Autodesk Fusion 360 part; units mm, degrees
note: some values were not read from the file. Chosen so that the rebuilt part matches the saved one: that a step has no effect.
(part 5 of 7)
  spline S1394 degree 3 poles (-52.4461, -9.6584) (-55.3128, -12.1512) (-55.3128, -12.1512) (-56.4346, -12.1512) knots 0 0 0 0 1 1 1 1
  spline S1395 degree 3 poles (-56.4346, -12.1512) (-56.0918, -10.9671) (-56.0918, -10.9671) (-55.4375, -9.6584) knots 0 0 0 0 1 1 1 1
  spline S1396 degree 3 poles (-55.4375, -9.6584) (-54.1287, -9.0041) (-54.1287, -9.0041) (-52.9447, -8.6613) knots 0 0 0 0 1 1 1 1
  spline S1397 degree 3 poles (11.369, -4.6729) (11.6981, -4.6729) (12.0271, -4.6729) (12.3662, -4.6729) knots 0 0 0 0 1 1 1 1
  spline S1398 degree 3 poles (12.3662, -4.6729) (12.2259, -5.4113) (12.0793, -6.1486) (11.9299, -6.8852) knots 0 0 0 0 1 1 1 1
  spline S1399 degree 3 poles (11.9299, -6.8852) (11.8489, -7.2959) (11.768, -7.7065) (11.6845, -8.1297) knots 0 0 0 0 1 1 1 1
  spline S1400 degree 3 poles (11.6845, -8.1297) (11.5284, -8.6396) (11.5284, -8.6396) (11.369, -9.1599) knots 0 0 0 0 1 1 1 1
  spline S1401 degree 3 poles (11.369, -9.1599) (10.8755, -9.4067) (10.8755, -9.4067) (10.3719, -9.6584) knots 0 0 0 0 1 1 1 1
  spline S1402 degree 3 poles (10.3719, -9.6584) (10.2825, -7.6905) (10.3253, -6.3689) (11.369, -4.6729) knots 0 0 0 0 1 1 1 1
  spline S1403 degree 3 poles (-34.4981, 8.2896) (-34.0045, 8.2896) (-33.511, 8.2896) (-33.0024, 8.2896) knots 0 0 0 0 1 1 1 1
  spline S1404 degree 3 poles (-33.0024, 8.2896) (-32.5039, 6.7939) (-32.5039, 6.7939) (-33.2206, 5.2048) knots 0 0 0 0 1 1 1 1
  spline S1405 degree 3 poles (-33.2206, 5.2048) (-33.6062, 4.5107) (-33.6062, 4.5107) (-33.9995, 3.8026) knots 0 0 0 0 1 1 1 1
  spline S1406 degree 3 poles (-33.9995, 3.8026) (-34.1641, 3.8026) (-34.3286, 3.8026) (-34.4981, 3.8026) knots 0 0 0 0 1 1 1 1
  spline S1407 degree 3 poles (-34.4981, 3.8026) (-34.9363, 6.8699) (-34.9363, 6.8699) (-34.9967, 7.791) knots 0 0 0 0 1 1 1 1
  spline S1408 degree 3 poles (-34.9967, 7.791) (-34.8321, 7.9556) (-34.6676, 8.1201) (-34.4981, 8.2896) knots 0 0 0 0 1 1 1 1
  spline S1409 degree 3 poles (-20.5385, 11.2809) (-20.374, 11.2809) (-20.2095, 11.2809) (-20.04, 11.2809) knots 0 0 0 0 1 1 1 1
  spline S1410 degree 3 poles (-20.04, 11.2809) (-20.04, 9.9647) (-20.04, 8.6485) (-20.04, 7.2925) knots 0 0 0 0 1 1 1 1
  spline S1411 degree 3 poles (-20.04, 7.2925) (-20.369, 7.2925) (-20.6981, 7.2925) (-21.0371, 7.2925) knots 0 0 0 0 1 1 1 1
  spline S1412 degree 3 poles (-21.0371, 7.2925) (-21.2016, 6.9634) (-21.3661, 6.6344) (-21.5356, 6.2954) knots 0 0 0 0 1 1 1 1
  spline S1413 degree 3 poles (-21.5356, 6.2954) (-21.7002, 6.9535) (-21.8647, 7.6116) (-22.0342, 8.2896) knots 0 0 0 0 1 1 1 1
  spline S1414 degree 3 poles (-22.0342, 8.2896) (-21.7052, 8.2896) (-21.3761, 8.2896) (-21.0371, 8.2896) knots 0 0 0 0 1 1 1 1
  spline S1415 degree 3 poles (-21.0371, 8.2896) (-21.0525, 8.8911) (-21.0525, 8.8911) (-21.0683, 9.5048) knots 0 0 0 0 1 1 1 1
  spline S1416 degree 3 poles (-21.0683, 9.5048) (-21.0371, 10.7824) (-21.0371, 10.7824) (-20.5385, 11.2809) knots 0 0 0 0 1 1 1 1
  spline S1417 degree 3 poles (0.8994, 35.2116) (1.0639, 35.2116) (1.2284, 35.2116) (1.3979, 35.2116) knots 0 0 0 0 1 1 1 1
  spline S1418 degree 3 poles (1.3979, 35.2116) (1.5624, 33.8954) (1.727, 32.5792) (1.8965, 31.2232) knots 0 0 0 0 1 1 1 1
  spline S1419 degree 3 poles (1.8965, 31.2232) (1.2384, 31.0586) (0.5803, 30.8941) (-0.0977, 30.7246) knots 0 0 0 0 1 1 1 1
  spline S1420 degree 3 poles (-0.0977, 30.7246) (0.2313, 32.2053) (0.5604, 33.686) (0.8994, 35.2116) knots 0 0 0 0 1 1 1 1
  spline S1421 degree 3 poles (31.3113, 37.2058) (31.4758, 36.7123) (31.6403, 36.2187) (31.8098, 35.7102) knots 0 0 0 0 1 1 1 1
  spline S1422 degree 3 poles (31.8098, 35.7102) (30.1808, 32.9014) (30.1808, 32.9014) (28.8185, 32.2203) knots 0 0 0 0 1 1 1 1
  spline S1423 degree 3 poles (28.8185, 32.2203) (29.0709, 34.0878) (29.3957, 34.9688) (30.8127, 36.2087) knots 0 0 0 0 1 1 1 1
  spline S1424 degree 3 poles (30.8127, 36.2087) (30.9773, 36.5378) (31.1418, 36.8668) (31.3113, 37.2058) knots 0 0 0 0 1 1 1 1
  spline S1425 degree 3 poles (-1.5934, 42.69) (-1.5934, 42.0319) (-1.5934, 41.3738) (-1.5934, 40.6957) knots 0 0 0 0 1 1 1 1
  spline S1426 degree 3 poles (-1.5934, 40.6957) (-1.9225, 40.6957) (-2.2515, 40.6957) (-2.5905, 40.6957) knots 0 0 0 0 1 1 1 1
  spline S1427 degree 3 poles (-2.5905, 40.6957) (-2.755, 40.2022) (-2.9196, 39.7086) (-3.0891, 39.2001) knots 0 0 0 0 1 1 1 1
  spline S1428 degree 3 poles (-3.0891, 39.2001) (-3.5876, 39.6986) (-3.5876, 39.6986) (-3.6188, 40.9762) knots 0 0 0 0 1 1 1 1
  spline S1429 degree 3 poles (-3.6188, 40.9762) (-3.6085, 41.3772) (-3.5982, 41.7782) (-3.5876, 42.1914) knots 0 0 0 0 1 1 1 1
  spline S1430 degree 3 poles (-3.5876, 42.1914) (-2.5905, 42.69) (-2.5905, 42.69) (-1.5934, 42.69) knots 0 0 0 0 1 1 1 1
  spline S1431 degree 3 poles (-77.3739, 6.2954) (-77.2094, 6.2954) (-77.0449, 6.2954) (-76.8754, 6.2954) knots 0 0 0 0 1 1 1 1
  spline S1432 degree 3 poles (-76.8754, 6.2954) (-77.0399, 4.4856) (-77.2044, 2.6758) (-77.3739, 0.8112) knots 0 0 0 0 1 1 1 1
  spline S1433 degree 3 poles (-77.3739, 0.8112) (-77.5384, 0.8112) (-77.703, 0.8112) (-77.8725, 0.8112) knots 0 0 0 0 1 1 1 1
  spline S1434 degree 3 poles (-77.8725, 0.8112) (-78.4861, 4.002) (-78.4861, 4.002) (-77.9036, 5.5164) knots 0 0 0 0 1 1 1 1
  spline S1435 degree 3 poles (-77.9036, 5.5164) (-77.7288, 5.7734) (-77.554, 6.0305) (-77.3739, 6.2954) knots 0 0 0 0 1 1 1 1
  spline S1436 degree 3 poles (-4.0862, 5.2983) (-3.5926, 5.2983) (-3.099, 5.2983) (-2.5905, 5.2983) knots 0 0 0 0 1 1 1 1
  spline S1437 degree 3 poles (-2.5905, 5.2983) (-2.7152, 4.1142) (-2.7152, 4.1142) (-3.0891, 2.8055) knots 0 0 0 0 1 1 1 1
  spline S1438 degree 3 poles (-3.0891, 2.8055) (-4.1173, 2.1511) (-4.1173, 2.1511) (-5.0833, 1.8084) knots 0 0 0 0 1 1 1 1
  spline S1439 degree 3 poles (-5.0833, 1.8084) (-4.7543, 2.96) (-4.4252, 4.1117) (-4.0862, 5.2983) knots 0 0 0 0 1 1 1 1
  spline S1440 degree 3 poles (18.3488, 14.7708) (18.1843, 13.9482) (18.0198, 13.1256) (17.8503, 12.278) knots 0 0 0 0 1 1 1 1
  spline S1441 degree 3 poles (17.8503, 12.278) (17.3567, 12.4426) (16.8631, 12.6071) (16.3546, 12.7766) knots 0 0 0 0 1 1 1 1
  spline S1442 degree 3 poles (16.3546, 12.7766) (16.1901, 13.2702) (16.0256, 13.7637) (15.8561, 14.2723) knots 0 0 0 0 1 1 1 1
  spline S1443 degree 3 poles (15.8561, 14.2723) (16.8532, 14.7708) (16.8532, 14.7708) (18.3488, 14.7708) knots 0 0 0 0 1 1 1 1
  spline S1444 degree 3 poles (-68.8985, 21.7506) (-68.5694, 21.7506) (-68.2404, 21.7506) (-67.9014, 21.7506) knots 0 0 0 0 1 1 1 1
  spline S1445 degree 3 poles (-67.9014, 21.7506) (-68.546, 20.3126) (-69.2272, 19.3215) (-70.3941, 18.2607) knots 0 0 0 0 1 1 1 1
  spline S1446 degree 3 poles (-70.3941, 18.2607) (-70.7232, 18.4252) (-71.0522, 18.5898) (-71.3913, 18.7593) knots 0 0 0 0 1 1 1 1
  spline S1447 degree 3 poles (-71.3913, 18.7593) (-70.5856, 19.7769) (-69.7532, 20.7738) (-68.8985, 21.7506) knots 0 0 0 0 1 1 1 1
  spline S1448 degree 3 poles (-7.5761, 35.2116) (-6.918, 35.0471) (-6.2599, 34.8826) (-5.5819, 34.7131) knots 0 0 0 0 1 1 1 1
  spline S1449 degree 3 poles (-5.5819, 34.7131) (-5.5819, 34.055) (-5.5819, 33.3969) (-5.5819, 32.7188) knots 0 0 0 0 1 1 1 1
  spline S1450 degree 3 poles (-5.5819, 32.7188) (-6.24, 32.7188) (-6.898, 32.7188) (-7.5761, 32.7188) knots 0 0 0 0 1 1 1 1
  spline S1451 degree 3 poles (-7.5761, 32.7188) (-7.5761, 33.5414) (-7.5761, 34.3641) (-7.5761, 35.2116) knots 0 0 0 0 1 1 1 1
  spline S1452 degree 3 poles (-45.9649, -7.6642) (-45.6358, -8.1578) (-45.3068, -8.6513) (-44.9678, -9.1599) knots 0 0 0 0 1 1 1 1
  spline S1453 degree 3 poles (-44.9678, -9.1599) (-45.4614, -9.4067) (-45.4614, -9.4067) (-45.9649, -9.6584) knots 0 0 0 0 1 1 1 1
  spline S1454 degree 3 poles (-45.9649, -9.6584) (-46.29, -10.6678) (-46.29, -10.6678) (-46.4635, -11.6527) knots 0 0 0 0 1 1 1 1
  spline S1455 degree 3 poles (-46.4635, -11.6527) (-46.957, -11.6527) (-47.4506, -11.6527) (-47.9591, -11.6527) knots 0 0 0 0 1 1 1 1
  spline S1456 degree 3 poles (-47.9591, -11.6527) (-47.3985, -10.171) (-46.8509, -8.9932) (-45.9649, -7.6642) knots 0 0 0 0 1 1 1 1
  spline S1457 degree 3 poles (-27.0198, -8.6613) (-26.5262, -8.6613) (-26.0326, -8.6613) (-25.5241, -8.6613) knots 0 0 0 0 1 1 1 1
  spline S1458 degree 3 poles (-25.5241, -8.6613) (-25.5241, -9.6485) (-25.5241, -10.6356) (-25.5241, -11.6527) knots 0 0 0 0 1 1 1 1
  spline S1459 degree 3 poles (-25.5241, -11.6527) (-26.0177, -11.6527) (-26.5112, -11.6527) (-27.0198, -11.6527) knots 0 0 0 0 1 1 1 1
  spline S1460 degree 3 poles (-27.0198, -11.6527) (-27.0198, -10.6655) (-27.0198, -9.6784) (-27.0198, -8.6613) knots 0 0 0 0 1 1 1 1
  spline S1461 degree 3 poles (32.3084, 31.7217) (33.2955, 31.4749) (33.2955, 31.4749) (34.3026, 31.2232) knots 0 0 0 0 1 1 1 1
  spline S1462 degree 3 poles (34.3026, 31.2232) (34.3026, 30.5651) (34.3026, 29.907) (34.3026, 29.2289) knots 0 0 0 0 1 1 1 1
  spline S1463 degree 3 poles (34.3026, 29.2289) (33.48, 29.3935) (32.6574, 29.558) (31.8098, 29.7275) knots 0 0 0 0 1 1 1 1
  spline S1464 degree 3 poles (31.8098, 29.7275) (32.3034, 30.2211) (32.797, 30.7146) (33.3055, 31.2232) knots 0 0 0 0 1 1 1 1
  spline S1465 degree 3 poles (33.3055, 31.2232) (32.9765, 31.3877) (32.6474, 31.5522) (32.3084, 31.7217) knots 0 0 0 0 1 1 1 1
sketch "Sketch84" plane through (76.6406, 0, 0) normal (1, 0, 0) x (0, 1, 0)
  line L0 (66.6352, 16.8343) -> (66.6352, 146.8343)
  line L1 (66.6352, 146.8343) -> (-58.3648, 111.8343)
  line L2 (-58.3648, 16.8343) -> (66.6352, 16.8343)
sketch "Sketch85" plane through (0, 0, 0) normal (1, 0, 0) x (0, 1, 0)
sketch "Sketch86" plane through (76.6406, 0, 0) normal (1, 0, 0) x (0, 1, 0)
sketch "Sketch87" plane through (76.6406, 0, 0) normal (1, 0, 0) x (0, 1, 0)
sketch "Sketch88" plane through (0, 0, 0) normal (0, 1, 0) x (1, 0, 0)
  line L0 (76.6406, -111.8343) -> (-103.3594, -111.8343)
  line L1 (-103.3594, -111.8343) -> (-103.3594, -16.8343)
  line L2 (-103.3594, -16.8343) -> (76.6406, -16.8343)
  line L3 (76.6406, -111.8343) -> (76.6406, -16.8343)
  line L4 (-103.3594, -111.8343) -> (76.6406, -111.8343)
  line L5 (76.6406, -111.8343) -> (76.6406, -16.8343)
  line L6 (76.6406, -16.8343) -> (-103.3594, -16.8343)
  line L7 (-103.3594, -16.8343) -> (-103.3594, -111.8343)
  constraint horizontal L4
  constraint vertical L5
  constraint horizontal L6
  constraint vertical L7
  constraint coincident L2.end L3.end
  constraint coincident L0.end L1.start
copy_body "Body->Comp1" bodies 1 removing the originals makes body 2 in component "Component"
sketch "Sketch89" plane through (-3.3594, 0, 0) normal (-1, 0, 0) x (0, -1, 0)
  line L0 (58.3648, 39.3343) -> (58.3648, 86.8343)
  line L1 (58.3648, 86.8343) -> (53.3648, 86.8343)
  line L2 (53.3648, 86.8343) -> (53.3648, 39.3343)
  line L3 (53.3648, 39.3343) -> (58.3648, 39.3343)
  line L4 (53.3648, 39.3343) -> (53.3648, 108.042)
  line L5 (58.3648, 111.8343) -> (58.3648, 16.8343)
  line L6 (58.3648, 39.3343) -> (53.3648, 39.3343)
  line L7 (57.3648, 39.3343) -> (54.3648, 39.3343)
  line L8 (54.3648, 39.3343) -> (54.3648, 64.7338)
  line L9 (54.3648, 64.7338) -> (57.3648, 64.7338)
  line L10 (57.3648, 64.7338) -> (57.3648, 39.3343)
  dimension "d135" = 3
  dimension "d136" = 1
  constraint horizontal L7
  constraint vertical L8
  constraint horizontal L9
  constraint vertical L10
  constraint coincident L3 L7.start
  measures "d135" distance of L7.start L7.end
  measures "d136" distance of L4 L8
extrude "Extrude1" cut sketch "Sketch89" along normal blind 95 and the other way blind 75 contours L3 L6 L7 L8 L9 L10 bodies 2 in component "Component"
sketch "Sketch90" plane through (-3.3594, 0, 0) normal (-1, 0, 0) x (0, -1, 0)
  line L0 (54.3648, 39.3343) -> (54.3648, 64.7338)
  line L1 (54.3648, 64.7338) -> (57.3648, 64.7338)
  line L2 (57.3648, 64.7338) -> (57.3648, 39.3343)
  line L3 (57.3648, 39.3343) -> (58.3648, 39.3343)
  line L4 (58.3648, 39.3343) -> (58.3648, 86.8343)
  line L5 (58.3648, 86.8343) -> (53.3648, 86.8343)
  line L6 (53.3648, 86.8343) -> (53.3648, 39.3343)
  line L7 (53.3648, 39.3343) -> (54.3648, 39.3343)
sketch "Sketch91" plane through (0, -58.3648, 0) normal (0, -1, 0) x (1, 0, 0)
  line L0 (-23.3594, 39.3343) -> (-23.3594, 86.8343)
  arc A0 (-3.3594, 86.8343) -> (-23.3594, 86.8343) centre (-13.3594, 86.8343) ccw
  line L1 (-3.3594, 86.8343) -> (-3.3594, 39.3343)
  line L2 (-3.3594, 39.3343) -> (71.6406, 39.3343)
  line L3 (71.6406, 39.3343) -> (71.6406, 16.8343)
  line L4 (71.6406, 16.8343) -> (76.6406, 16.8343)
  line L5 (76.6406, 16.8343) -> (76.6406, 111.8343)
  line L6 (76.6406, 111.8343) -> (-103.3594, 111.8343)
  line L7 (-103.3594, 111.8343) -> (-103.3594, 16.8343)
  line L8 (-103.3594, 16.8343) -> (-98.3594, 16.8343)
  line L9 (-98.3594, 16.8343) -> (-98.3594, 39.3343)
  line L10 (-98.3594, 39.3343) -> (-23.3594, 39.3343)
  line L11 (7, 75) -> (-31, 75)
  line L12 (-31, 75) -> (-31, 101)
  line L13 (-31, 101) -> (7, 101)
  line L14 (7, 101) -> (7, 75)
  constraint horizontal L11
  constraint vertical L12
  constraint horizontal L13
  constraint vertical L14
extrude "Extrude2" add sketch "Sketch91" against normal blind 5 contours L0 A0 L1 L11 bodies 2 in component "Component"
sketch "Sketch92" plane through (-3.3594, 0, 0) normal (-1, 0, 0) x (0, -1, 0)
  line L0 (53.3648, 86.8343) -> (53.3648, 39.3343)
  line L1 (58.3648, 111.8343) -> (58.3648, 16.8343)
  line L2 (57.3648, 64.3343) -> (54.3648, 64.3343)
  line L3 (54.3648, 64.3343) -> (54.3648, 91)
  line L4 (54.3648, 91) -> (57.3648, 91)
  line L5 (57.3648, 91) -> (57.3648, 64.3343)
  dimension "d143" = 3
  dimension "d144" = 1
  constraint horizontal L2
  constraint vertical L3
  constraint horizontal L4
  constraint vertical L5
  measures "d143" distance of L2.start L2.end
  measures "d144" distance of L0 L3
extrude "Extrude3" cut sketch "Sketch92" along normal blind 95 and the other way blind 75 bodies 2 in component "Component"
sketch "Sketch93" plane through (0, -58.3648, 0) normal (0, -1, 0) x (1, 0, 0)
  line L0 (-23.3594, 39.3343) -> (-23.3594, 75)
  line L1 (-23.3594, 75) -> (-3.3594, 75)
  line L2 (-3.3594, 75) -> (-3.3594, 39.3343)
  line L3 (-3.3594, 39.3343) -> (71.6406, 39.3343)
  line L4 (71.6406, 39.3343) -> (71.6406, 16.8343)
  line L5 (71.6406, 16.8343) -> (76.6406, 16.8343)
  line L6 (76.6406, 16.8343) -> (76.6406, 111.8343)
  line L7 (76.6406, 111.8343) -> (-103.3594, 111.8343)
  line L8 (-103.3594, 111.8343) -> (-103.3594, 16.8343)
  line L9 (-103.3594, 16.8343) -> (-98.3594, 16.8343)
  line L10 (-98.3594, 16.8343) -> (-98.3594, 39.3343)
  line L11 (-98.3594, 39.3343) -> (-23.3594, 39.3343)
  line L12 (-3.3594, 39.3343) -> (-3.3594, 86.8343)
  line L13 (-3.3594, 75) -> (-23.3594, 75)
  line L14 (-23.3594, 39.3343) -> (-23.3594, 75)
  line L15 (-98.3594, 39.3343) -> (-23.3594, 39.3343)
  line L16 (-3.3594, 39.3343) -> (71.6406, 39.3343)
  line L17 (-98.3594, 16.8343) -> (-98.3594, 39.3343)
  line L18 (71.6406, 21.8343) -> (-98.3594, 21.8343)
  line L19 (71.6406, 16.8343) -> (71.6406, 39.3343)
  line L20 (-23.3594, 75) -> (-3.3594, 75)
  line L21 (-3.3594, 75) -> (-3.3594, 39.3343)
  line L22 (-3.3594, 39.3343) -> (-23.3594, 39.3343)
  line L23 (-23.3594, 39.3343) -> (-23.3594, 75)
  line L24 (-98.3594, 39.3343) -> (71.6406, 39.3343)
  line L25 (71.6406, 39.3343) -> (71.6406, 18.7368)
  line L26 (71.6406, 18.7368) -> (-98.3594, 18.7368)
  line L27 (-98.3594, 18.7368) -> (-98.3594, 39.3343)
  constraint horizontal L20
  constraint vertical L21
  constraint horizontal L22
  constraint vertical L23
  constraint coincident L2.end L3.start
  constraint coincident L0.end L1.start
  constraint horizontal L24
  constraint vertical L25
  constraint horizontal L26
  constraint vertical L27
  constraint coincident L19 L25.end
  constraint coincident L10.end L11.start
sketch "Sketch94" plane through (0, -61.3648, 0) normal (0, -1, 0) x (1, 0, 0)
sketch "Sketch95" plane through (0, -61.3648, 0) normal (0, -1, 0) x (1, 0, 0)
  line L0 (-23.3594, 75) -> (-23.3594, 39.3343)
  line L1 (-3.3594, 39.3343) -> (-3.3594, 75)
  line L2 (-3.3594, 71.6642) -> (-23.3594, 71.6642)
  line L3 (-23.3594, 71.6642) -> (-23.3594, 81.6642)
  line L4 (-23.3594, 81.6642) -> (-3.3594, 81.6642)
  line L5 (-3.3594, 81.6642) -> (-3.3594, 71.6642)
  dimension "d151" = 20
  dimension "d152" = 10
  constraint horizontal L2
  constraint vertical L3
  constraint horizontal L4
  constraint vertical L5
  constraint coincident L1 L2.start
  measures "d151" distance of L2.start L2.end
  measures "d152" distance of L2.start L4.end
sketch "Sketch96" plane through (0, 0, 0) normal (1, 0, 0) x (0, 1, 0)
fillet "Fillet1" radius 5 1 edges at (-13.3594, 66.6352, 146.8343) on bodies 2 in component "Component"
fillet "Fillet2'" radius 7.5 1 edges at (-13.3594, -58.3648, 111.8343) on bodies 2 in component "Component"
sketch "Sketch97" plane through (0, -58.3648, 0) normal (0, -1, 0) x (1, 0, 0)
  line L0 (76.6406, 106.1458) -> (-103.3594, 106.1458)
  line L1 (-103.3594, 106.1458) -> (-103.3594, 16.8343)
  line L2 (-103.3594, 16.8343) -> (-98.3594, 16.8343)
  line L3 (-98.3594, 16.8343) -> (-98.3594, 39.3343)
  line L4 (-98.3594, 39.3343) -> (-23.3594, 39.3343)
  line L5 (-23.3594, 39.3343) -> (-23.3594, 75)
  line L6 (-23.3594, 75) -> (-3.3594, 75)
  line L7 (-3.3594, 39.3343) -> (71.6406, 39.3343)
  line L8 (71.6406, 16.8343) -> (76.6406, 16.8343)
  line L9 (76.6406, 16.8343) -> (76.6406, 106.1458)
sketch "Sketch98" plane through (71.6406, 0, 0) normal (-1, 0, 0) x (0, -1, 0)
  arc A0 (-60.2871, 145.0568) -> (-61.6142, 145.2419) centre (-61.6352, 140.242) ccw
  arc A1 (-61.6142, 145.2419) -> (10.7755, 21.8343) centre (112.3399, 164.3463) ccw
  line L0 (10.7755, 21.8343) -> (46.1173, 21.8343)
  arc A2 (58.3648, 16.8343) -> (46.1173, 21.8343) centre (46.1173, 4.3343) ccw
  line L1 (58.3648, 16.8343) -> (58.3648, 39.3343)
  line L2 (58.3648, 39.3343) -> (57.3648, 39.3343)
  line L3 (57.3648, 39.3343) -> (57.3648, 91)
  line L4 (57.3648, 91) -> (54.3648, 91)
  line L5 (54.3648, 91) -> (54.3648, 39.3343)
  line L6 (54.3648, 39.3343) -> (53.3648, 39.3343)
  line L7 (53.3648, 39.3343) -> (53.3648, 108.042)
  line L8 (53.3648, 108.042) -> (-27.8352, 130.778)
  line L9 (-27.8352, 130.778) -> (-26.4871, 135.5928)
  line L10 (-26.4871, 135.5928) -> (-60.2871, 145.0568)
sketch "Sketch99" plane through (71.6406, 0, 0) normal (-1, 0, 0) x (0, -1, 0)
sketch "Sketch100" plane through (-103.3594, 0, 0) normal (-1, 0, 0) x (0, -1, 0)
  arc A0 (58.3648, 106.1458) -> (52.887, 113.3681) centre (50.8648, 106.1458) ccw
  line L0 (52.887, 113.3681) -> (-60.2871, 145.0568)
  arc A1 (-60.2871, 145.0568) -> (-66.6352, 140.242) centre (-61.6352, 140.242) ccw
  line L1 (-66.6352, 140.242) -> (-66.6352, 16.8343)
  line L2 (-66.6352, 16.8343) -> (58.3648, 16.8343)
  line L3 (58.3648, 16.8343) -> (58.3648, 106.1458)
  spline S0 degree 3 poles (2.2852, 67.0349) (2.2852, 66.9197) (2.2852, 66.8045) (2.2852, 66.6858) knots 0 0 0 0 1 1 1 1
  spline S1 degree 3 poles (2.2852, 66.6858) (2.3869, 66.6426) (2.4886, 66.5994) (2.5934, 66.5549) knots 0 0 0 0 1 1 1 1
  spline S2 degree 3 poles (2.5934, 66.5549) (3.0411, 66.3044) (3.304, 66.0266) (3.6379, 65.6385) knots 0 0 0 0 1 1 1 1
  spline S3 degree 3 poles (3.6379, 65.6385) (3.7985, 65.4549) (3.7985, 65.4549) (3.9624, 65.2676) knots 0 0 0 0 1 1 1 1
  spline S4 degree 3 poles (3.9624, 65.2676) (4.2052, 64.9404) (4.2052, 64.9404) (4.2052, 64.5913) knots 0 0 0 0 1 1 1 1
  spline S5 degree 3 poles (4.2052, 64.5913) (4.3204, 64.5913) (4.4356, 64.5913) (4.5543, 64.5913) knots 0 0 0 0 1 1 1 1
  spline S6 degree 3 poles (4.5543, 64.5913) (4.8188, 64.3165) (4.8188, 64.3165) (5.1215, 63.9476) knots 0 0 0 0 1 1 1 1
  spline S7 degree 3 poles (5.1215, 63.9476) (5.5144, 63.4823) (5.8983, 63.071) (6.3761, 62.6931) knots 0 0 0 0 1 1 1 1
  spline S8 degree 3 poles (6.3761, 62.6931) (6.5237, 62.5707) (6.6713, 62.4483) (6.8233, 62.3222) knots 0 0 0 0 1 1 1 1
  spline S9 degree 3 poles (6.8233, 62.3222) (6.8233, 62.207) (6.8233, 62.0918) (6.8233, 61.9731) knots 0 0 0 0 1 1 1 1
  spline S10 degree 3 poles (6.8233, 61.9731) (6.9385, 61.9731) (7.0537, 61.9731) (7.1724, 61.9731) knots 0 0 0 0 1 1 1 1
  spline S11 degree 3 poles (7.1724, 61.9731) (7.1724, 61.8579) (7.1724, 61.7427) (7.1724, 61.624) knots 0 0 0 0 1 1 1 1
  spline S12 degree 3 poles (7.1724, 61.624) (7.2876, 61.624) (7.4028, 61.624) (7.5215, 61.624) knots 0 0 0 0 1 1 1 1
  spline S13 degree 3 poles (7.5215, 61.624) (7.5215, 61.5088) (7.5215, 61.3936) (7.5215, 61.2749) knots 0 0 0 0 1 1 1 1
  spline S14 degree 3 poles (7.5215, 61.2749) (7.6196, 61.2299) (7.7177, 61.1849) (7.8188, 61.1385) knots 0 0 0 0 1 1 1 1
  spline S15 degree 3 poles (7.8188, 61.1385) (8.2663, 60.9011) (8.6477, 60.6242) (9.0488, 60.3149) knots 0 0 0 0 1 1 1 1
  spline S16 degree 3 poles (9.0488, 60.3149) (9.258, 60.1556) (9.258, 60.1556) (9.4715, 59.9931) knots 0 0 0 0 1 1 1 1
  spline S17 degree 3 poles (9.4715, 59.9931) (9.5768, 59.8977) (9.6821, 59.8023) (9.7906, 59.704) knots 0 0 0 0 1 1 1 1
  spline S18 degree 3 poles (9.7906, 59.704) (9.7906, 59.5888) (9.7906, 59.4736) (9.7906, 59.3549) knots 0 0 0 0 1 1 1 1
  spline S19 degree 3 poles (9.7906, 59.3549) (9.9368, 59.2877) (9.9368, 59.2877) (10.0858, 59.2192) knots 0 0 0 0 1 1 1 1
  spline S20 degree 3 poles (10.0858, 59.2192) (10.5426, 58.9773) (10.9359, 58.6927) (11.3506, 58.384) knots 0 0 0 0 1 1 1 1
  spline S21 degree 3 poles (11.3506, 58.384) (12.893, 57.2537) (14.3989, 56.1754) (16.0852, 55.2749) knots 0 0 0 0 1 1 1 1
  spline S22 degree 3 poles (16.0852, 55.2749) (17.4185, 54.5565) (18.5489, 53.6736) (19.5651, 52.5476) knots 0 0 0 0 1 1 1 1
  spline S23 degree 3 poles (19.5651, 52.5476) (19.5651, 52.4324) (19.5651, 52.3172) (19.5651, 52.1986) knots 0 0 0 0 1 1 1 1
  spline S24 degree 3 poles (19.5651, 52.1986) (19.6803, 52.1986) (19.7955, 52.1986) (19.9142, 52.1986) knots 0 0 0 0 1 1 1 1
  spline S25 degree 3 poles (19.9142, 52.1986) (20.2033, 51.7772) (20.2033, 51.7772) (20.5251, 51.2167) knots 0 0 0 0 1 1 1 1
  spline S26 degree 3 poles (20.5251, 51.2167) (20.6313, 51.0345) (20.7375, 50.8522) (20.847, 50.6645) knots 0 0 0 0 1 1 1 1
  spline S27 degree 3 poles (20.847, 50.6645) (22.0278, 48.3752) (22.0625, 45.7608) (21.4851, 43.2967) knots 0 0 0 0 1 1 1 1
  spline S28 degree 3 poles (21.4851, 43.2967) (21.0727, 42.0296) (20.5204, 40.8165) (19.9142, 39.6313) knots 0 0 0 0 1 1 1 1
  spline S29 degree 3 poles (19.9142, 39.6313) (19.799, 39.6313) (19.6838, 39.6313) (19.5651, 39.6313) knots 0 0 0 0 1 1 1 1
  spline S30 degree 3 poles (19.5651, 39.6313) (19.5492, 39.5332) (19.5332, 39.4351) (19.5167, 39.334) knots 0 0 0 0 1 1 1 1
  spline S31 degree 3 poles (19.5167, 39.334) (19.0996, 38.0083) (17.6464, 36.6724) (16.5979, 35.7913) knots 0 0 0 0 1 1 1 1
  spline S32 degree 3 poles (16.5979, 35.7913) (16.4827, 35.7913) (16.3675, 35.7913) (16.2488, 35.7913) knots 0 0 0 0 1 1 1 1
  spline S33 degree 3 poles (16.2488, 35.7913) (16.2488, 35.6761) (16.2488, 35.5609) (16.2488, 35.4422) knots 0 0 0 0 1 1 1 1
  spline S34 degree 3 poles (16.2488, 35.4422) (15.3247, 34.744) (15.3247, 34.744) (14.6779, 34.744) knots 0 0 0 0 1 1 1 1
  spline S35 degree 3 poles (14.6779, 34.744) (14.6779, 34.6288) (14.6779, 34.5136) (14.6779, 34.3949) knots 0 0 0 0 1 1 1 1
  spline S36 degree 3 poles (14.6779, 34.3949) (13.2065, 33.5376) (11.8044, 32.8829) (10.1397, 32.4749) knots 0 0 0 0 1 1 1 1
  spline S37 degree 3 poles (10.1397, 32.4749) (10.0283, 32.4457) (9.9169, 32.4164) (9.8022, 32.3863) knots 0 0 0 0 1 1 1 1
  spline S38 degree 3 poles (9.8022, 32.3863) (8.3795, 32.0527) (6.9553, 32.0741) (5.5033, 32.0751) knots 0 0 0 0 1 1 1 1
  spline S39 degree 3 poles (5.5033, 32.0751) (5.2138, 32.0741) (4.9243, 32.0729) (4.6348, 32.0716) knots 0 0 0 0 1 1 1 1
  spline S40 degree 3 poles (4.6348, 32.0716) (3.8525, 32.0685) (3.0703, 32.0677) (2.288, 32.0675) knots 0 0 0 0 1 1 1 1
  spline S41 degree 3 poles (2.288, 32.0675) (1.7977, 32.0672) (1.3075, 32.0665) (0.8173, 32.0655) knots 0 0 0 0 1 1 1 1
  spline S42 degree 3 poles (0.8173, 32.0655) (-0.8973, 32.0623) (-2.6119, 32.0609) (-4.3265, 32.0612) knots 0 0 0 0 1 1 1 1
  spline S43 degree 3 poles (-4.3265, 32.0612) (-5.9177, 32.0614) (-7.5087, 32.0577) (-9.0999, 32.0522) knots 0 0 0 0 1 1 1 1
  spline S44 degree 3 poles (-9.0999, 32.0522) (-10.4715, 32.0476) (-11.8432, 32.0457) (-13.2149, 32.046) knots 0 0 0 0 1 1 1 1
  spline S45 degree 3 poles (-13.2149, 32.046) (-14.0316, 32.0461) (-14.8483, 32.0451) (-15.665, 32.0414) knots 0 0 0 0 1 1 1 1
  spline S46 degree 3 poles (-15.665, 32.0414) (-16.4345, 32.0379) (-17.204, 32.038) (-17.9735, 32.0405) knots 0 0 0 0 1 1 1 1
  spline S47 degree 3 poles (-17.9735, 32.0405) (-18.2534, 32.0409) (-18.5334, 32.0401) (-18.8133, 32.0379) knots 0 0 0 0 1 1 1 1
  spline S48 degree 3 poles (-18.8133, 32.0379) (-22.1905, 32.0139) (-25.1526, 32.8254) (-28.0421, 34.6022) knots 0 0 0 0 1 1 1 1
  spline S49 degree 3 poles (-28.0421, 34.6022) (-28.2297, 34.7175) (-28.2297, 34.7175) (-28.4212, 34.8351) knots 0 0 0 0 1 1 1 1
  spline S50 degree 3 poles (-28.4212, 34.8351) (-28.7234, 35.0272) (-29.0165, 35.2335) (-29.3075, 35.4422) knots 0 0 0 0 1 1 1 1
  spline S51 degree 3 poles (-29.3075, 35.4422) (-29.3075, 35.5574) (-29.3075, 35.6726) (-29.3075, 35.7913) knots 0 0 0 0 1 1 1 1
  spline S52 degree 3 poles (-29.3075, 35.7913) (-29.4106, 35.8377) (-29.5136, 35.884) (-29.6198, 35.9318) knots 0 0 0 0 1 1 1 1
  spline S53 degree 3 poles (-29.6198, 35.9318) (-30.7043, 36.5181) (-31.6521, 37.7094) (-32.2748, 38.7586) knots 0 0 0 0 1 1 1 1
  spline S54 degree 3 poles (-32.2748, 38.7586) (-32.2748, 38.9314) (-32.2748, 39.1042) (-32.2748, 39.2822) knots 0 0 0 0 1 1 1 1
  spline S55 degree 3 poles (-32.2748, 39.2822) (-32.39, 39.2822) (-32.5052, 39.2822) (-32.6239, 39.2822) knots 0 0 0 0 1 1 1 1
  spline S56 degree 3 poles (-32.6239, 39.2822) (-34.3047, 42.2909) (-34.9525, 45.5857) (-34.1075, 48.9695) knots 0 0 0 0 1 1 1 1
  spline S57 degree 3 poles (-34.1075, 48.9695) (-33.69, 50.2235) (-33.0248, 51.2919) (-32.2748, 52.3731) knots 0 0 0 0 1 1 1 1
  spline S58 degree 3 poles (-32.2748, 52.3731) (-32.1347, 52.5776) (-32.1347, 52.5776) (-31.9918, 52.7863) knots 0 0 0 0 1 1 1 1
  spline S59 degree 3 poles (-31.9918, 52.7863) (-31.9124, 52.8803) (-31.833, 52.9744) (-31.7511, 53.0713) knots 0 0 0 0 1 1 1 1
  spline S60 degree 3 poles (-31.7511, 53.0713) (-31.6359, 53.0713) (-31.5207, 53.0713) (-31.4021, 53.0713) knots 0 0 0 0 1 1 1 1
  spline S61 degree 3 poles (-31.4021, 53.0713) (-31.4021, 53.1865) (-31.4021, 53.3017) (-31.4021, 53.4204) knots 0 0 0 0 1 1 1 1
  spline S62 degree 3 poles (-31.4021, 53.4204) (-31.2869, 53.4204) (-31.1717, 53.4204) (-31.053, 53.4204) knots 0 0 0 0 1 1 1 1
  spline S63 degree 3 poles (-31.053, 53.4204) (-31.053, 53.5356) (-31.053, 53.6508) (-31.053, 53.7695) knots 0 0 0 0 1 1 1 1
  spline S64 degree 3 poles (-31.053, 53.7695) (-30.9378, 53.7695) (-30.8226, 53.7695) (-30.7039, 53.7695) knots 0 0 0 0 1 1 1 1
  spline S65 degree 3 poles (-30.7039, 53.7695) (-30.7039, 53.8847) (-30.7039, 53.9999) (-30.7039, 54.1186) knots 0 0 0 0 1 1 1 1
  spline S66 degree 3 poles (-30.7039, 54.1186) (-30.5887, 54.1186) (-30.4735, 54.1186) (-30.3548, 54.1186) knots 0 0 0 0 1 1 1 1
  spline S67 degree 3 poles (-30.3548, 54.1186) (-30.3548, 54.2338) (-30.3548, 54.349) (-30.3548, 54.4676) knots 0 0 0 0 1 1 1 1
  spline S68 degree 3 poles (-30.3548, 54.4676) (-30.0141, 54.7084) (-29.6742, 54.9275) (-29.3184, 55.144) knots 0 0 0 0 1 1 1 1
  spline S69 degree 3 poles (-29.3184, 55.144) (-28.3429, 55.7547) (-27.389, 56.3886) (-26.4493, 57.0531) knots 0 0 0 0 1 1 1 1
  spline S70 degree 3 poles (-26.4493, 57.0531) (-26.3266, 57.1399) (-26.2039, 57.2266) (-26.0774, 57.316) knots 0 0 0 0 1 1 1 1
  spline S71 degree 3 poles (-26.0774, 57.316) (-25.0435, 58.0524) (-24.0285, 58.8133) (-23.024, 59.5893) knots 0 0 0 0 1 1 1 1
  spline S72 degree 3 poles (-23.024, 59.5893) (-22.1885, 60.2276) (-22.1885, 60.2276) (-21.8021, 60.2276) knots 0 0 0 0 1 1 1 1
  spline S73 degree 3 poles (-21.8021, 60.2276) (-21.8021, 60.3428) (-21.8021, 60.458) (-21.8021, 60.5767) knots 0 0 0 0 1 1 1 1
  spline S74 degree 3 poles (-21.8021, 60.5767) (-21.5141, 60.6919) (-21.2261, 60.8071) (-20.9293, 60.9258) knots 0 0 0 0 1 1 1 1
  spline S75 degree 3 poles (-20.9293, 60.9258) (-20.9293, 61.041) (-20.9293, 61.1562) (-20.9293, 61.2749) knots 0 0 0 0 1 1 1 1
  spline S76 degree 3 poles (-20.9293, 61.2749) (-20.6362, 61.5763) (-20.6362, 61.5763) (-20.253, 61.9076) knots 0 0 0 0 1 1 1 1
  spline S77 degree 3 poles (-20.253, 61.9076) (-20.1274, 62.0179) (-20.0019, 62.1281) (-19.8725, 62.2417) knots 0 0 0 0 1 1 1 1
  spline S78 degree 3 poles (-19.8725, 62.2417) (-19.533, 62.4967) (-19.533, 62.4967) (-19.1839, 62.4967) knots 0 0 0 0 1 1 1 1
  spline S79 degree 3 poles (-19.1839, 62.4967) (-19.1839, 62.6119) (-19.1839, 62.7271) (-19.1839, 62.8458) knots 0 0 0 0 1 1 1 1
  spline S80 degree 3 poles (-19.1839, 62.8458) (-18.9439, 63.1294) (-18.9439, 63.1294) (-18.6603, 63.3694) knots 0 0 0 0 1 1 1 1
  spline S81 degree 3 poles (-18.6603, 63.3694) (-18.5451, 63.3694) (-18.4299, 63.3694) (-18.3112, 63.3694) knots 0 0 0 0 1 1 1 1
  spline S82 degree 3 poles (-18.3112, 63.3694) (-18.3112, 63.4846) (-18.3112, 63.5998) (-18.3112, 63.7185) knots 0 0 0 0 1 1 1 1
  spline S83 degree 3 poles (-18.3112, 63.7185) (-18.196, 63.7185) (-18.0808, 63.7185) (-17.9621, 63.7185) knots 0 0 0 0 1 1 1 1
  spline S84 degree 3 poles (-17.9621, 63.7185) (-17.9621, 63.8337) (-17.9621, 63.9489) (-17.9621, 64.0676) knots 0 0 0 0 1 1 1 1
  spline S85 degree 3 poles (-17.9621, 64.0676) (-17.8469, 64.0676) (-17.7317, 64.0676) (-17.613, 64.0676) knots 0 0 0 0 1 1 1 1
  spline S86 degree 3 poles (-17.613, 64.0676) (-17.5734, 64.1576) (-17.5338, 64.2476) (-17.493, 64.3404) knots 0 0 0 0 1 1 1 1
  spline S87 degree 3 poles (-17.493, 64.3404) (-17.1797, 64.9221) (-16.8276, 65.4897) (-16.3912, 65.9876) knots 0 0 0 0 1 1 1 1
  spline S88 degree 3 poles (-16.3912, 65.9876) (-16.276, 65.9876) (-16.1608, 65.9876) (-16.0421, 65.9876) knots 0 0 0 0 1 1 1 1
  spline S89 degree 3 poles (-16.0421, 65.9876) (-16.0421, 66.1028) (-16.0421, 66.218) (-16.0421, 66.3367) knots 0 0 0 0 1 1 1 1
  spline S90 degree 3 poles (-16.0421, 66.3367) (-15.9269, 66.3367) (-15.8117, 66.3367) (-15.693, 66.3367) knots 0 0 0 0 1 1 1 1
  spline S91 degree 3 poles (-15.693, 66.3367) (-15.693, 66.4519) (-15.693, 66.5671) (-15.693, 66.6858) knots 0 0 0 0 1 1 1 1
  spline S92 degree 3 poles (-15.693, 66.6858) (-15.5778, 66.6858) (-15.4626, 66.6858) (-15.3439, 66.6858) knots 0 0 0 0 1 1 1 1
  spline S93 degree 3 poles (-15.3439, 66.6858) (-15.2575, 66.945) (-15.2575, 66.945) (-15.1694, 67.2094) knots 0 0 0 0 1 1 1 1
  spline S94 degree 3 poles (-15.1694, 67.2094) (-14.8094, 67.3294) (-14.8094, 67.3294) (-14.4712, 67.384) knots 0 0 0 0 1 1 1 1
  spline S95 degree 3 poles (-14.4712, 67.384) (-14.4712, 67.4992) (-14.4712, 67.6144) (-14.4712, 67.7331) knots 0 0 0 0 1 1 1 1
  spline S96 degree 3 poles (-14.4712, 67.7331) (-14.2984, 67.7331) (-14.1256, 67.7331) (-13.9475, 67.7331) knots 0 0 0 0 1 1 1 1
  spline S97 degree 3 poles (-13.9475, 67.7331) (-13.9475, 67.8483) (-13.9475, 67.9635) (-13.9475, 68.0822) knots 0 0 0 0 1 1 1 1
  spline S98 degree 3 poles (-13.9475, 68.0822) (-8.5843, 70.5951) (-2.6424, 70.6367) (2.2852, 67.0349) knots 0 0 0 0 1 1 1 1
  spline S99 degree 3 poles (-14.4582, 101.8301) (-13.8382, 101.3962) (-13.2407, 100.9292) (-12.7257, 100.373) knots 0 0 0 0 1 1 1 1
  spline S100 degree 3 poles (-12.7257, 100.373) (-12.7257, 100.2578) (-12.7257, 100.1426) (-12.7257, 100.0239) knots 0 0 0 0 1 1 1 1
  spline S101 degree 3 poles (-12.7257, 100.0239) (-12.6238, 99.9812) (-12.5219, 99.9384) (-12.4169, 99.8944) knots 0 0 0 0 1 1 1 1
  spline S102 degree 3 poles (-12.4169, 99.8944) (-10.2033, 98.6461) (-8.7919, 94.8938) (-8.1153, 92.5627) knots 0 0 0 0 1 1 1 1
  spline S103 degree 3 poles (-8.1153, 92.5627) (-6.8362, 87.6435) (-7.5634, 82.927) (-10.1075, 78.5549) knots 0 0 0 0 1 1 1 1
  spline S104 degree 3 poles (-10.1075, 78.5549) (-10.1933, 78.4057) (-10.279, 78.2565) (-10.3673, 78.1028) knots 0 0 0 0 1 1 1 1
  spline S105 degree 3 poles (-10.3673, 78.1028) (-10.5594, 77.7804) (-10.7679, 77.4679) (-10.9803, 77.1585) knots 0 0 0 0 1 1 1 1
  spline S106 degree 3 poles (-10.9803, 77.1585) (-11.0955, 77.1585) (-11.2107, 77.1585) (-11.3294, 77.1585) knots 0 0 0 0 1 1 1 1
  spline S107 degree 3 poles (-11.3294, 77.1585) (-11.3726, 77.0577) (-11.4158, 76.9569) (-11.4603, 76.8531) knots 0 0 0 0 1 1 1 1
  spline S108 degree 3 poles (-11.4603, 76.8531) (-11.7104, 76.4028) (-11.9899, 76.1006) (-12.3766, 75.7622) knots 0 0 0 0 1 1 1 1
  spline S109 degree 3 poles (-12.3766, 75.7622) (-12.4918, 75.7622) (-12.607, 75.7622) (-12.7257, 75.7622) knots 0 0 0 0 1 1 1 1
  spline S110 degree 3 poles (-12.7257, 75.7622) (-12.7814, 75.6106) (-12.7814, 75.6106) (-12.8382, 75.456) knots 0 0 0 0 1 1 1 1
  spline S111 degree 3 poles (-12.8382, 75.456) (-13.6328, 74.1394) (-15.8719, 73.364) (-17.2605, 72.9435) knots 0 0 0 0 1 1 1 1
  spline S112 degree 3 poles (-17.2605, 72.9435) (-19.9437, 72.3065) (-22.3674, 72.9502) (-24.7693, 74.1913) knots 0 0 0 0 1 1 1 1
  spline S113 degree 3 poles (-24.7693, 74.1913) (-24.7693, 74.3065) (-24.7693, 74.4217) (-24.7693, 74.5403) knots 0 0 0 0 1 1 1 1
  spline S114 degree 3 poles (-24.7693, 74.5403) (-24.9691, 74.6159) (-24.9691, 74.6159) (-25.173, 74.6931) knots 0 0 0 0 1 1 1 1
  spline S115 degree 3 poles (-25.173, 74.6931) (-25.6421, 74.8894) (-25.6421, 74.8894) (-26.1657, 75.2385) knots 0 0 0 0 1 1 1 1
  spline S116 degree 3 poles (-26.1657, 75.2385) (-26.1657, 75.3537) (-26.1657, 75.4689) (-26.1657, 75.5876) knots 0 0 0 0 1 1 1 1
  spline S117 degree 3 poles (-26.1657, 75.5876) (-26.3206, 75.6511) (-26.3206, 75.6511) (-26.4787, 75.7158) knots 0 0 0 0 1 1 1 1
  spline S118 degree 3 poles (-26.4787, 75.7158) (-28.101, 76.6461) (-29.1243, 79.3828) (-29.6408, 81.1246) knots 0 0 0 0 1 1 1 1
  spline S119 degree 3 poles (-29.6408, 81.1246) (-30.8847, 85.9011) (-29.782, 90.6076) (-27.3875, 94.7876) knots 0 0 0 0 1 1 1 1
  spline S120 degree 3 poles (-27.3875, 94.7876) (-27.2723, 94.7876) (-27.1571, 94.7876) (-27.0384, 94.7876) knots 0 0 0 0 1 1 1 1
  spline S121 degree 3 poles (-27.0384, 94.7876) (-26.9574, 94.9928) (-26.9574, 94.9928) (-26.8748, 95.2021) knots 0 0 0 0 1 1 1 1
  spline S122 degree 3 poles (-26.8748, 95.2021) (-26.6893, 95.6603) (-26.6893, 95.6603) (-26.5148, 96.0094) knots 0 0 0 0 1 1 1 1
  spline S123 degree 3 poles (-26.5148, 96.0094) (-26.3996, 96.0094) (-26.2844, 96.0094) (-26.1657, 96.0094) knots 0 0 0 0 1 1 1 1
  spline S124 degree 3 poles (-26.1657, 96.0094) (-26.1657, 96.1246) (-26.1657, 96.2398) (-26.1657, 96.3585) knots 0 0 0 0 1 1 1 1
  spline S125 degree 3 poles (-26.1657, 96.3585) (-26.0505, 96.3585) (-25.9353, 96.3585) (-25.8166, 96.3585) knots 0 0 0 0 1 1 1 1
  spline S126 degree 3 poles (-25.8166, 96.3585) (-25.8166, 96.4737) (-25.8166, 96.5889) (-25.8166, 96.7076) knots 0 0 0 0 1 1 1 1
  spline S127 degree 3 poles (-25.8166, 96.7076) (-25.7014, 96.7076) (-25.5862, 96.7076) (-25.4675, 96.7076) knots 0 0 0 0 1 1 1 1
  spline S128 degree 3 poles (-25.4675, 96.7076) (-25.42, 96.8097) (-25.3726, 96.9119) (-25.3237, 97.0171) knots 0 0 0 0 1 1 1 1
  spline S129 degree 3 poles (-25.3237, 97.0171) (-24.9079, 97.8044) (-24.37, 98.4782) (-23.5693, 98.8785) knots 0 0 0 0 1 1 1 1
  spline S130 degree 3 poles (-23.5693, 98.8785) (-23.4469, 98.9109) (-23.3245, 98.9433) (-23.1984, 98.9767) knots 0 0 0 0 1 1 1 1
  spline S131 degree 3 poles (-23.1984, 98.9767) (-23.1984, 99.0919) (-23.1984, 99.2071) (-23.1984, 99.3258) knots 0 0 0 0 1 1 1 1
  spline S132 degree 3 poles (-23.1984, 99.3258) (-21.1735, 101.2521) (-17.1515, 103.3858) (-14.4582, 101.8301) knots 0 0 0 0 1 1 1 1
  spline S133 degree 3 poles (9.7906, 101.9439) (10.9269, 101.2858) (12.1392, 100.5705) (13.107, 99.6749) knots 0 0 0 0 1 1 1 1
  spline S134 degree 3 poles (13.107, 99.6749) (13.107, 99.5597) (13.107, 99.4445) (13.107, 99.3258) knots 0 0 0 0 1 1 1 1
  spline S135 degree 3 poles (13.107, 99.3258) (13.2114, 99.279) (13.3158, 99.2322) (13.4233, 99.1839) knots 0 0 0 0 1 1 1 1
  spline S136 degree 3 poles (13.4233, 99.1839) (13.8049, 98.9768) (14.0518, 98.7854) (14.3288, 98.453) knots 0 0 0 0 1 1 1 1
  spline S137 degree 3 poles (14.3288, 98.453) (14.3288, 98.3378) (14.3288, 98.2226) (14.3288, 98.1039) knots 0 0 0 0 1 1 1 1
  spline S138 degree 3 poles (14.3288, 98.1039) (14.444, 98.1039) (14.5592, 98.1039) (14.6779, 98.1039) knots 0 0 0 0 1 1 1 1
  spline S139 degree 3 poles (14.6779, 98.1039) (14.6779, 97.9887) (14.6779, 97.8735) (14.6779, 97.7549) knots 0 0 0 0 1 1 1 1
  spline S140 degree 3 poles (14.6779, 97.7549) (14.7931, 97.7549) (14.9083, 97.7549) (15.027, 97.7549) knots 0 0 0 0 1 1 1 1
  spline S141 degree 3 poles (15.027, 97.7549) (15.5506, 97.1507) (15.5506, 97.1507) (15.5506, 96.7076) knots 0 0 0 0 1 1 1 1
  spline S142 degree 3 poles (15.5506, 96.7076) (15.6658, 96.7076) (15.781, 96.7076) (15.8997, 96.7076) knots 0 0 0 0 1 1 1 1
  spline S143 degree 3 poles (15.8997, 96.7076) (16.1531, 96.3793) (16.3908, 96.0388) (16.6197, 95.693) knots 0 0 0 0 1 1 1 1
  spline S144 degree 3 poles (16.6197, 95.693) (16.8094, 95.4106) (16.8094, 95.4106) (17.0029, 95.1224) knots 0 0 0 0 1 1 1 1
  spline S145 degree 3 poles (17.0029, 95.1224) (17.2961, 94.613) (17.2961, 94.613) (17.2961, 94.0894) knots 0 0 0 0 1 1 1 1
  spline S146 degree 3 poles (17.2961, 94.0894) (17.4113, 94.0894) (17.5265, 94.0894) (17.6451, 94.0894) knots 0 0 0 0 1 1 1 1
  spline S147 degree 3 poles (17.6451, 94.0894) (18.8718, 91.6602) (19.6619, 89.3415) (19.7397, 86.584) knots 0 0 0 0 1 1 1 1
  spline S148 degree 3 poles (19.7397, 86.584) (19.7446, 86.4229) (19.7496, 86.2618) (19.7547, 86.0958) knots 0 0 0 0 1 1 1 1
  spline S149 degree 3 poles (19.7547, 86.0958) (19.7616, 85.6175) (19.7537, 85.1421) (19.7397, 84.664) knots 0 0 0 0 1 1 1 1
  spline S150 degree 3 poles (19.7397, 84.664) (19.7353, 84.4038) (19.7353, 84.4038) (19.7308, 84.1383) knots 0 0 0 0 1 1 1 1
  spline S151 degree 3 poles (19.7308, 84.1383) (19.6087, 81.3021) (18.5084, 78.2374) (16.5979, 76.1112) knots 0 0 0 0 1 1 1 1
  spline S152 degree 3 poles (16.5979, 76.1112) (16.3132, 75.8709) (16.0242, 75.6352) (15.7252, 75.4131) knots 0 0 0 0 1 1 1 1
  spline S153 degree 3 poles (15.7252, 75.4131) (15.6676, 75.2979) (15.61, 75.1827) (15.5506, 75.064) knots 0 0 0 0 1 1 1 1
  spline S154 degree 3 poles (15.5506, 75.064) (13.0011, 73.4176) (10.2473, 72.7277) (7.2488, 73.3403) knots 0 0 0 0 1 1 1 1
  spline S155 degree 3 poles (7.2488, 73.3403) (5.0371, 73.9132) (3.1266, 75.1229) (1.587, 76.8094) knots 0 0 0 0 1 1 1 1
  spline S156 degree 3 poles (1.587, 76.8094) (1.587, 76.9246) (1.587, 77.0398) (1.587, 77.1585) knots 0 0 0 0 1 1 1 1
  spline S157 degree 3 poles (1.587, 77.1585) (1.4142, 77.2161) (1.2414, 77.2737) (1.0634, 77.3331) knots 0 0 0 0 1 1 1 1
  spline S158 degree 3 poles (1.0634, 77.3331) (-1.7395, 80.7779) (-2.9058, 85.3366) (-2.6021, 89.7258) knots 0 0 0 0 1 1 1 1
  spline S159 degree 3 poles (-2.6021, 89.7258) (-2.2684, 92.9181) (-1.0461, 96.3347) (1.0634, 98.8021) knots 0 0 0 0 1 1 1 1
  spline S160 degree 3 poles (1.0634, 98.8021) (1.2362, 98.8597) (1.409, 98.9173) (1.587, 98.9767) knots 0 0 0 0 1 1 1 1
  spline S161 degree 3 poles (1.587, 98.9767) (1.715, 99.3284) (1.715, 99.3284) (1.7615, 99.6749) knots 0 0 0 0 1 1 1 1
  spline S162 degree 3 poles (1.7615, 99.6749) (1.8767, 99.6749) (1.9919, 99.6749) (2.1106, 99.6749) knots 0 0 0 0 1 1 1 1
  spline S163 degree 3 poles (2.1106, 99.6749) (2.1106, 99.7901) (2.1106, 99.9053) (2.1106, 100.0239) knots 0 0 0 0 1 1 1 1
  spline S164 degree 3 poles (2.1106, 100.0239) (2.2258, 100.0239) (2.341, 100.0239) (2.4597, 100.0239) knots 0 0 0 0 1 1 1 1
  spline S165 degree 3 poles (2.4597, 100.0239) (2.4597, 100.1391) (2.4597, 100.2543) (2.4597, 100.373) knots 0 0 0 0 1 1 1 1
  spline S166 degree 3 poles (2.4597, 100.373) (4.7401, 102.3417) (6.8952, 103.4843) (9.7906, 101.9439) knots 0 0 0 0 1 1 1 1
  spline S167 degree 3 poles (-35.2093, 80.8676) (-35.0473, 80.738) (-34.8853, 80.6084) (-34.7184, 80.4749) knots 0 0 0 0 1 1 1 1
  spline S168 degree 3 poles (-34.7184, 80.4749) (-34.7184, 80.3597) (-34.7184, 80.2445) (-34.7184, 80.1258) knots 0 0 0 0 1 1 1 1
  spline S169 degree 3 poles (-34.7184, 80.1258) (-34.614, 80.0754) (-34.5096, 80.025) (-34.4021, 79.9731) knots 0 0 0 0 1 1 1 1
  spline S170 degree 3 poles (-34.4021, 79.9731) (-34.0202, 79.7767) (-34.0202, 79.7767) (-33.4966, 79.4276) knots 0 0 0 0 1 1 1 1
  spline S171 degree 3 poles (-33.4966, 79.4276) (-33.4966, 79.3124) (-33.4966, 79.1972) (-33.4966, 79.0785) knots 0 0 0 0 1 1 1 1
  spline S172 degree 3 poles (-33.4966, 79.0785) (-33.3814, 79.0785) (-33.2662, 79.0785) (-33.1475, 79.0785) knots 0 0 0 0 1 1 1 1
  spline S173 degree 3 poles (-33.1475, 79.0785) (-33.1475, 78.9633) (-33.1475, 78.8481) (-33.1475, 78.7294) knots 0 0 0 0 1 1 1 1
  spline S174 degree 3 poles (-33.1475, 78.7294) (-33.0323, 78.7294) (-32.9171, 78.7294) (-32.7984, 78.7294) knots 0 0 0 0 1 1 1 1
  spline S175 degree 3 poles (-32.7984, 78.7294) (-32.7984, 78.6142) (-32.7984, 78.499) (-32.7984, 78.3803) knots 0 0 0 0 1 1 1 1
  spline S176 degree 3 poles (-32.7984, 78.3803) (-32.6832, 78.3803) (-32.568, 78.3803) (-32.4493, 78.3803) knots 0 0 0 0 1 1 1 1
  spline S177 degree 3 poles (-32.4493, 78.3803) (-32.2765, 77.9483) (-32.2765, 77.9483) (-32.1002, 77.5076) knots 0 0 0 0 1 1 1 1
  spline S178 degree 3 poles (-32.1002, 77.5076) (-31.985, 77.5076) (-31.8698, 77.5076) (-31.7511, 77.5076) knots 0 0 0 0 1 1 1 1
  spline S179 degree 3 poles (-31.7511, 77.5076) (-31.2275, 76.9034) (-31.2275, 76.9034) (-31.2275, 76.4603) knots 0 0 0 0 1 1 1 1
  spline S180 degree 3 poles (-31.2275, 76.4603) (-31.1123, 76.4603) (-30.9971, 76.4603) (-30.8784, 76.4603) knots 0 0 0 0 1 1 1 1
  spline S181 degree 3 poles (-30.8784, 76.4603) (-30.5184, 75.826) (-30.1725, 75.185) (-29.8312, 74.5403) knots 0 0 0 0 1 1 1 1
  spline S182 degree 3 poles (-29.8312, 74.5403) (-29.7265, 74.3444) (-29.6219, 74.1484) (-29.5141, 73.9465) knots 0 0 0 0 1 1 1 1
  spline S183 degree 3 poles (-29.5141, 73.9465) (-27.9126, 70.8241) (-27.2376, 66.9016) (-28.2602, 63.4894) knots 0 0 0 0 1 1 1 1
  spline S184 degree 3 poles (-28.2602, 63.4894) (-28.3715, 63.1568) (-28.4857, 62.825) (-28.6093, 62.4967) knots 0 0 0 0 1 1 1 1
  spline S185 degree 3 poles (-28.6093, 62.4967) (-28.7245, 62.4967) (-28.8397, 62.4967) (-28.9584, 62.4967) knots 0 0 0 0 1 1 1 1
  spline S186 degree 3 poles (-28.9584, 62.4967) (-29.0052, 62.3419) (-29.052, 62.1871) (-29.1002, 62.0276) knots 0 0 0 0 1 1 1 1
  spline S187 degree 3 poles (-29.1002, 62.0276) (-29.2944, 61.4859) (-29.4999, 61.0461) (-29.8312, 60.5767) knots 0 0 0 0 1 1 1 1
  spline S188 degree 3 poles (-29.8312, 60.5767) (-29.9464, 60.5767) (-30.0616, 60.5767) (-30.1802, 60.5767) knots 0 0 0 0 1 1 1 1
  spline S189 degree 3 poles (-30.1802, 60.5767) (-30.2954, 60.3463) (-30.4106, 60.1159) (-30.5293, 59.8785) knots 0 0 0 0 1 1 1 1
  spline S190 degree 3 poles (-30.5293, 59.8785) (-30.6445, 59.8785) (-30.7597, 59.8785) (-30.8784, 59.8785) knots 0 0 0 0 1 1 1 1
  spline S191 degree 3 poles (-30.8784, 59.8785) (-30.8784, 59.7633) (-30.8784, 59.6481) (-30.8784, 59.5295) knots 0 0 0 0 1 1 1 1
  spline S192 degree 3 poles (-30.8784, 59.5295) (-30.9936, 59.5295) (-31.1088, 59.5295) (-31.2275, 59.5295) knots 0 0 0 0 1 1 1 1
  spline S193 degree 3 poles (-31.2275, 59.5295) (-31.2275, 59.4143) (-31.2275, 59.2991) (-31.2275, 59.1804) knots 0 0 0 0 1 1 1 1
  spline S194 degree 3 poles (-31.2275, 59.1804) (-33.4674, 57.4514) (-36.0912, 56.6269) (-38.9075, 56.9113) knots 0 0 0 0 1 1 1 1
  spline S195 degree 3 poles (-38.9075, 56.9113) (-39.5978, 57.0628) (-40.1959, 57.2951) (-40.8275, 57.6095) knots 0 0 0 0 1 1 1 1
  spline S196 degree 3 poles (-40.8275, 57.6095) (-40.974, 57.6815) (-41.1204, 57.7535) (-41.2714, 57.8276) knots 0 0 0 0 1 1 1 1
  spline S197 degree 3 poles (-41.2714, 57.8276) (-42.6681, 58.5899) (-44.1572, 59.719) (-44.6675, 61.2749) knots 0 0 0 0 1 1 1 1
  spline S198 degree 3 poles (-44.6675, 61.2749) (-44.7827, 61.2749) (-44.8979, 61.2749) (-45.0166, 61.2749) knots 0 0 0 0 1 1 1 1
  spline S199 degree 3 poles (-45.0166, 61.2749) (-45.1367, 61.5152) (-45.1367, 61.5152) (-45.2593, 61.7604) knots 0 0 0 0 1 1 1 1
  spline S200 degree 3 poles (-45.2593, 61.7604) (-45.3367, 61.915) (-45.3367, 61.915) (-45.4156, 62.0727) knots 0 0 0 0 1 1 1 1
  spline S201 degree 3 poles (-45.4156, 62.0727) (-45.5286, 62.2988) (-45.6413, 62.525) (-45.7538, 62.7513) knots 0 0 0 0 1 1 1 1
  spline S202 degree 3 poles (-45.7538, 62.7513) (-45.9811, 63.2079) (-46.2085, 63.663) (-46.4504, 64.1119) knots 0 0 0 0 1 1 1 1
  spline S203 degree 3 poles (-46.4504, 64.1119) (-48.3195, 67.5873) (-48.54, 72.1388) (-47.5223, 75.9033) knots 0 0 0 0 1 1 1 1
  spline S204 degree 3 poles (-47.5223, 75.9033) (-47.1499, 77.1241) (-46.6199, 78.2812) (-46.0639, 79.4276) knots 0 0 0 0 1 1 1 1
  spline S205 degree 3 poles (-46.0639, 79.4276) (-45.9487, 79.4276) (-45.8335, 79.4276) (-45.7148, 79.4276) knots 0 0 0 0 1 1 1 1
  spline S206 degree 3 poles (-45.7148, 79.4276) (-45.5996, 79.7732) (-45.4844, 80.1188) (-45.3657, 80.4749) knots 0 0 0 0 1 1 1 1
  spline S207 degree 3 poles (-45.3657, 80.4749) (-45.2505, 80.4749) (-45.1353, 80.4749) (-45.0166, 80.4749) knots 0 0 0 0 1 1 1 1
  spline S208 degree 3 poles (-45.0166, 80.4749) (-44.9878, 80.5973) (-44.959, 80.7197) (-44.9293, 80.8458) knots 0 0 0 0 1 1 1 1
  spline S209 degree 3 poles (-44.9293, 80.8458) (-44.5534, 81.5662) (-43.9706, 81.9918) (-43.2711, 82.3949) knots 0 0 0 0 1 1 1 1
  spline S210 degree 3 poles (-43.2711, 82.3949) (-43.0983, 82.3949) (-42.9255, 82.3949) (-42.7475, 82.3949) knots 0 0 0 0 1 1 1 1
  spline S211 degree 3 poles (-42.7475, 82.3949) (-42.7475, 82.5101) (-42.7475, 82.6253) (-42.7475, 82.744) knots 0 0 0 0 1 1 1 1
  spline S212 degree 3 poles (-42.7475, 82.744) (-40.0163, 83.6038) (-37.4647, 82.4045) (-35.2093, 80.8676) knots 0 0 0 0 1 1 1 1
  spline S213 degree 3 poles (31.2597, 82.3949) (31.2597, 82.2797) (31.2597, 82.1645) (31.2597, 82.0458) knots 0 0 0 0 1 1 1 1
  spline S214 degree 3 poles (31.2597, 82.0458) (31.4129, 82.0147) (31.4129, 82.0147) (31.5692, 81.9831) knots 0 0 0 0 1 1 1 1
  spline S215 degree 3 poles (31.5692, 81.9831) (32.203, 81.8007) (32.6946, 81.4396) (33.1797, 80.9985) knots 0 0 0 0 1 1 1 1
  spline S216 degree 3 poles (33.1797, 80.9985) (33.4306, 80.5076) (33.4306, 80.5076) (33.5288, 80.1258) knots 0 0 0 0 1 1 1 1
  spline S217 degree 3 poles (33.5288, 80.1258) (33.644, 80.1258) (33.7592, 80.1258) (33.8779, 80.1258) knots 0 0 0 0 1 1 1 1
  spline S218 degree 3 poles (33.8779, 80.1258) (33.8779, 80.0106) (33.8779, 79.8954) (33.8779, 79.7767) knots 0 0 0 0 1 1 1 1
  spline S219 degree 3 poles (33.8779, 79.7767) (33.9931, 79.7767) (34.1083, 79.7767) (34.2269, 79.7767) knots 0 0 0 0 1 1 1 1
  spline S220 degree 3 poles (34.2269, 79.7767) (36.5375, 75.6542) (37.6913, 71.1669) (36.456, 66.4678) knots 0 0 0 0 1 1 1 1
  spline S221 degree 3 poles (36.456, 66.4678) (35.7778, 64.1019) (34.8484, 61.76) (33.2697, 59.8506) knots 0 0 0 0 1 1 1 1
  spline S222 degree 3 poles (33.2697, 59.8506) (32.9769, 59.5062) (32.9769, 59.5062) (32.656, 59.0058) knots 0 0 0 0 1 1 1 1
  spline S223 degree 3 poles (32.656, 59.0058) (32.5408, 59.0058) (32.4256, 59.0058) (32.3069, 59.0058) knots 0 0 0 0 1 1 1 1
  spline S224 degree 3 poles (32.3069, 59.0058) (32.3069, 58.8906) (32.3069, 58.7754) (32.3069, 58.6567) knots 0 0 0 0 1 1 1 1
  spline S225 degree 3 poles (32.3069, 58.6567) (32.1917, 58.6567) (32.0765, 58.6567) (31.9579, 58.6567) knots 0 0 0 0 1 1 1 1
  spline S226 degree 3 poles (31.9579, 58.6567) (31.9579, 58.5415) (31.9579, 58.4263) (31.9579, 58.3076) knots 0 0 0 0 1 1 1 1
  spline S227 degree 3 poles (31.9579, 58.3076) (30.1404, 56.7711) (28.0036, 56.2387) (25.6742, 56.3876) knots 0 0 0 0 1 1 1 1
  spline S228 degree 3 poles (25.6742, 56.3876) (23.6581, 56.6779) (21.7225, 57.6294) (20.0888, 58.8313) knots 0 0 0 0 1 1 1 1
  spline S229 degree 3 poles (20.0888, 58.8313) (20.0888, 58.9465) (20.0888, 59.0617) (20.0888, 59.1804) knots 0 0 0 0 1 1 1 1
  spline S230 degree 3 poles (20.0888, 59.1804) (19.9736, 59.1804) (19.8584, 59.1804) (19.7397, 59.1804) knots 0 0 0 0 1 1 1 1
  spline S231 degree 3 poles (19.7397, 59.1804) (19.7397, 59.2956) (19.7397, 59.4108) (19.7397, 59.5295) knots 0 0 0 0 1 1 1 1
  spline S232 degree 3 poles (19.7397, 59.5295) (19.6245, 59.5295) (19.5093, 59.5295) (19.3906, 59.5295) knots 0 0 0 0 1 1 1 1
  spline S233 degree 3 poles (19.3906, 59.5295) (19.3906, 59.6447) (19.3906, 59.7599) (19.3906, 59.8785) knots 0 0 0 0 1 1 1 1
  spline S234 degree 3 poles (19.3906, 59.8785) (19.2754, 59.8785) (19.1602, 59.8785) (19.0415, 59.8785) knots 0 0 0 0 1 1 1 1
  spline S235 degree 3 poles (19.0415, 59.8785) (16.9736, 62.797) (16.65, 65.899) (17.1699, 69.3558) knots 0 0 0 0 1 1 1 1
  spline S236 degree 3 poles (17.1699, 69.3558) (17.7978, 72.5733) (19.2026, 75.4212) (21.3106, 77.9112) knots 0 0 0 0 1 1 1 1
  spline S237 degree 3 poles (21.3106, 77.9112) (21.3955, 78.0116) (21.4803, 78.1119) (21.5677, 78.2153) knots 0 0 0 0 1 1 1 1
  spline S238 degree 3 poles (21.5677, 78.2153) (22.1754, 78.9139) (22.8225, 79.5875) (23.5797, 80.1258) knots 0 0 0 0 1 1 1 1
  spline S239 degree 3 poles (23.5797, 80.1258) (23.6949, 80.1258) (23.8101, 80.1258) (23.9288, 80.1258) knots 0 0 0 0 1 1 1 1
  spline S240 degree 3 poles (23.9288, 80.1258) (23.9288, 80.241) (23.9288, 80.3562) (23.9288, 80.4749) knots 0 0 0 0 1 1 1 1
  spline S241 degree 3 poles (23.9288, 80.4749) (26.1446, 82.1286) (28.5077, 83.3122) (31.2597, 82.3949) knots 0 0 0 0 1 1 1 1
  spline S242 degree 3 poles (23.5797, 80.1258) (23.6949, 80.0682) (23.8101, 80.0106) (23.9288, 79.9512) knots 0 0 0 0 1 1 1 1